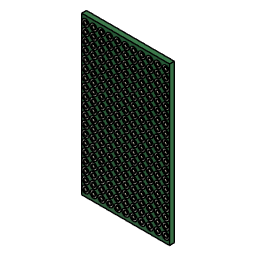
pcb_daughterboard (Autodesk Fusion 360 design; units mm, degrees)
Autodesk Fusion 360 part; units mm, degrees
(part 1 of 2)
sketch "PCB Daughterboard" plane through (0, 0, 0) normal (0, 1, 0) x (1, 0, 0)
  line L0 (0, 0) -> (38, 0)
  line L1 (38, 0) -> (38, -65)
  line L2 (38, -65) -> (0, -65)
  line L3 (0, -65) -> (0, 0)
  dimension "d3" = 38
  dimension "d4" = 65
  constraint horizontal L0
  constraint vertical L1
  constraint horizontal L2
  constraint vertical L3
  constraint coincident L0.start L3.end
  measures "d3" distance of L0.start L0.end
  measures "d4" distance of L0.end L1.end
extrude "Extrude1" add sketch "PCB Daughterboard" along normal blind 1.5 makes body 1
sketch "Holes" plane through (0, 0, 0) normal (0, -1, 0) x (1, 0, 0)
  line L0 (38, 65) -> (0, 65)
  line L1 (0, 65) -> (0, 0)
  line L2 (0, 0) -> (38, 0)
  line L3 (38, 0) -> (38, 65)
  circle A0 centre (1.22, 62.975) radius 0.6
  dimension "d5" = 1.2
  dimension "d12" = 1.22
  dimension "d13" = 2.025
  measures "d5" diameter of A0
  measures "d12" distance of L1 A0.centre
  measures "d13" distance of L0 A0.centre
extrude "Extrude2" cut sketch "Holes" against normal blind 1.5 contours A0 bodies 1
pattern_linear "R-Pattern1" count 19 spacing 2.5396 along (0, 0, -1) count 11 spacing 2.54 along (1, 0, 0) of "Extrude2"
sketch "Condutive Metal" plane through (0, 0, 0) normal (0, -1, 0) x (1, 0, 0)
  circle A0 centre (26.62, 17.262) radius 0.6
  circle A1 centre (26.62, 19.8016) radius 0.6
  circle A2 centre (26.62, 22.3412) radius 0.6
  circle A3 centre (26.62, 24.8808) radius 0.6
  circle A4 centre (26.62, 27.4204) radius 0.6
  circle A5 centre (26.62, 29.9601) radius 0.6
  circle A6 centre (26.62, 32.4997) radius 0.6
  circle A7 centre (26.62, 35.0393) radius 0.6
  circle A8 centre (26.62, 37.5789) radius 0.6
  circle A9 centre (26.62, 40.1185) radius 0.6
  circle A10 centre (26.62, 42.6581) radius 0.6
  circle A11 centre (26.62, 45.1977) radius 0.6
  circle A12 centre (26.62, 47.7373) radius 0.6
  circle A13 centre (26.62, 50.2769) radius 0.6
  circle A14 centre (26.62, 52.8166) radius 0.6
  circle A15 centre (26.62, 55.3562) radius 0.6
  circle A16 centre (26.62, 57.8958) radius 0.6
  circle A17 centre (26.62, 60.4354) radius 0.6
  circle A18 centre (26.62, 62.975) radius 0.6
  circle A19 centre (24.08, 17.262) radius 0.6
  circle A20 centre (24.08, 19.8016) radius 0.6
  circle A21 centre (24.08, 22.3412) radius 0.6
  circle A22 centre (24.08, 24.8808) radius 0.6
  circle A23 centre (24.08, 27.4204) radius 0.6
  circle A24 centre (24.08, 29.9601) radius 0.6
  circle A25 centre (24.08, 32.4997) radius 0.6
  circle A26 centre (24.08, 35.0393) radius 0.6
  circle A27 centre (24.08, 37.5789) radius 0.6
  circle A28 centre (24.08, 40.1185) radius 0.6
  circle A29 centre (24.08, 42.6581) radius 0.6
  circle A30 centre (24.08, 45.1977) radius 0.6
  circle A31 centre (24.08, 47.7373) radius 0.6
  circle A32 centre (24.08, 50.2769) radius 0.6
  circle A33 centre (24.08, 52.8166) radius 0.6
  circle A34 centre (24.08, 55.3562) radius 0.6
  circle A35 centre (24.08, 57.8958) radius 0.6
  circle A36 centre (24.08, 60.4354) radius 0.6
  circle A37 centre (24.08, 62.975) radius 0.6
  circle A38 centre (21.54, 17.262) radius 0.6
  circle A39 centre (21.54, 19.8016) radius 0.6
  circle A40 centre (21.54, 22.3412) radius 0.6
  circle A41 centre (21.54, 24.8808) radius 0.6
  circle A42 centre (21.54, 27.4204) radius 0.6
  circle A43 centre (21.54, 29.9601) radius 0.6
  circle A44 centre (21.54, 32.4997) radius 0.6
  circle A45 centre (21.54, 35.0393) radius 0.6
  circle A46 centre (21.54, 37.5789) radius 0.6
  circle A47 centre (21.54, 40.1185) radius 0.6
  circle A48 centre (21.54, 42.6581) radius 0.6
  circle A49 centre (21.54, 45.1977) radius 0.6
  circle A50 centre (21.54, 47.7373) radius 0.6
  circle A51 centre (21.54, 50.2769) radius 0.6
  circle A52 centre (21.54, 52.8166) radius 0.6
  circle A53 centre (21.54, 55.3562) radius 0.6
  circle A54 centre (21.54, 57.8958) radius 0.6
  circle A55 centre (21.54, 60.4354) radius 0.6
  circle A56 centre (21.54, 62.975) radius 0.6
  circle A57 centre (19, 17.262) radius 0.6
  circle A58 centre (19, 19.8016) radius 0.6
  circle A59 centre (19, 22.3412) radius 0.6
  circle A60 centre (19, 24.8808) radius 0.6
  circle A61 centre (19, 27.4204) radius 0.6
  circle A62 centre (19, 29.9601) radius 0.6
  circle A63 centre (19, 32.4997) radius 0.6
  circle A64 centre (19, 35.0393) radius 0.6
  circle A65 centre (19, 37.5789) radius 0.6
  circle A66 centre (19, 40.1185) radius 0.6
  circle A67 centre (19, 42.6581) radius 0.6
  circle A68 centre (19, 45.1977) radius 0.6
  circle A69 centre (19, 47.7373) radius 0.6
  circle A70 centre (19, 50.2769) radius 0.6
  circle A71 centre (19, 52.8166) radius 0.6
  circle A72 centre (19, 55.3562) radius 0.6
  circle A73 centre (19, 57.8958) radius 0.6
  circle A74 centre (19, 60.4354) radius 0.6
  circle A75 centre (19, 62.975) radius 0.6
  circle A76 centre (16.46, 17.262) radius 0.6
  circle A77 centre (16.46, 19.8016) radius 0.6
  circle A78 centre (16.46, 22.3412) radius 0.6
  circle A79 centre (16.46, 24.8808) radius 0.6
  circle A80 centre (16.46, 27.4204) radius 0.6
  circle A81 centre (16.46, 29.9601) radius 0.6
  circle A82 centre (16.46, 32.4997) radius 0.6
  circle A83 centre (16.46, 35.0393) radius 0.6
  circle A84 centre (16.46, 37.5789) radius 0.6
  circle A85 centre (16.46, 40.1185) radius 0.6
  circle A86 centre (16.46, 42.6581) radius 0.6
  circle A87 centre (16.46, 45.1977) radius 0.6
  circle A88 centre (16.46, 47.7373) radius 0.6
  circle A89 centre (16.46, 50.2769) radius 0.6
  circle A90 centre (16.46, 52.8166) radius 0.6
  circle A91 centre (16.46, 55.3562) radius 0.6
  circle A92 centre (16.46, 57.8958) radius 0.6
  circle A93 centre (16.46, 60.4354) radius 0.6
  circle A94 centre (16.46, 62.975) radius 0.6
  circle A95 centre (13.92, 17.262) radius 0.6
  circle A96 centre (13.92, 19.8016) radius 0.6
  circle A97 centre (13.92, 22.3412) radius 0.6
  circle A98 centre (13.92, 24.8808) radius 0.6
  circle A99 centre (13.92, 27.4204) radius 0.6
  circle A100 centre (13.92, 29.9601) radius 0.6
  circle A101 centre (13.92, 32.4997) radius 0.6
  circle A102 centre (13.92, 35.0393) radius 0.6
  circle A103 centre (13.92, 37.5789) radius 0.6
  circle A104 centre (13.92, 40.1185) radius 0.6
  circle A105 centre (13.92, 42.6581) radius 0.6
  circle A106 centre (13.92, 45.1977) radius 0.6
  circle A107 centre (13.92, 47.7373) radius 0.6
  circle A108 centre (13.92, 50.2769) radius 0.6
  circle A109 centre (13.92, 52.8166) radius 0.6
  circle A110 centre (13.92, 55.3562) radius 0.6
  circle A111 centre (13.92, 57.8958) radius 0.6
  circle A112 centre (13.92, 60.4354) radius 0.6
  circle A113 centre (13.92, 62.975) radius 0.6
  circle A114 centre (11.38, 17.262) radius 0.6
  circle A115 centre (11.38, 19.8016) radius 0.6
  circle A116 centre (11.38, 22.3412) radius 0.6
  circle A117 centre (11.38, 24.8808) radius 0.6
  circle A118 centre (11.38, 27.4204) radius 0.6
  circle A119 centre (11.38, 29.9601) radius 0.6
  circle A120 centre (11.38, 32.4997) radius 0.6
  circle A121 centre (11.38, 35.0393) radius 0.6
  circle A122 centre (11.38, 37.5789) radius 0.6
  circle A123 centre (11.38, 40.1185) radius 0.6
  circle A124 centre (11.38, 42.6581) radius 0.6
  circle A125 centre (11.38, 45.1977) radius 0.6
  circle A126 centre (11.38, 47.7373) radius 0.6
  circle A127 centre (11.38, 50.2769) radius 0.6
  circle A128 centre (11.38, 52.8166) radius 0.6
  circle A129 centre (11.38, 55.3562) radius 0.6
  circle A130 centre (11.38, 57.8958) radius 0.6
  circle A131 centre (11.38, 60.4354) radius 0.6
  circle A132 centre (11.38, 62.975) radius 0.6
  circle A133 centre (8.84, 17.262) radius 0.6
  circle A134 centre (8.84, 19.8016) radius 0.6
  circle A135 centre (8.84, 22.3412) radius 0.6
  circle A136 centre (8.84, 24.8808) radius 0.6
  circle A137 centre (8.84, 27.4204) radius 0.6
  circle A138 centre (8.84, 29.9601) radius 0.6
  circle A139 centre (8.84, 32.4997) radius 0.6
  circle A140 centre (8.84, 35.0393) radius 0.6
  circle A141 centre (8.84, 37.5789) radius 0.6
  circle A142 centre (8.84, 40.1185) radius 0.6
  circle A143 centre (8.84, 42.6581) radius 0.6
  circle A144 centre (8.84, 45.1977) radius 0.6
  circle A145 centre (8.84, 47.7373) radius 0.6
  circle A146 centre (8.84, 50.2769) radius 0.6
  circle A147 centre (8.84, 52.8166) radius 0.6
  circle A148 centre (8.84, 55.3562) radius 0.6
  circle A149 centre (8.84, 57.8958) radius 0.6
  circle A150 centre (8.84, 60.4354) radius 0.6
  circle A151 centre (8.84, 62.975) radius 0.6
  circle A152 centre (6.3, 17.262) radius 0.6
  circle A153 centre (6.3, 19.8016) radius 0.6
  circle A154 centre (6.3, 22.3412) radius 0.6
  circle A155 centre (6.3, 24.8808) radius 0.6
  circle A156 centre (6.3, 27.4204) radius 0.6
  circle A157 centre (6.3, 29.9601) radius 0.6
  circle A158 centre (6.3, 32.4997) radius 0.6
  circle A159 centre (6.3, 35.0393) radius 0.6
  circle A160 centre (6.3, 37.5789) radius 0.6
  circle A161 centre (6.3, 40.1185) radius 0.6
  circle A162 centre (6.3, 42.6581) radius 0.6
  circle A163 centre (6.3, 45.1977) radius 0.6
  circle A164 centre (6.3, 47.7373) radius 0.6
  circle A165 centre (6.3, 50.2769) radius 0.6
  circle A166 centre (6.3, 52.8166) radius 0.6
  circle A167 centre (6.3, 55.3562) radius 0.6
  circle A168 centre (6.3, 57.8958) radius 0.6
  circle A169 centre (6.3, 60.4354) radius 0.6
  circle A170 centre (6.3, 62.975) radius 0.6
  circle A171 centre (3.76, 17.262) radius 0.6
  circle A172 centre (3.76, 19.8016) radius 0.6
  circle A173 centre (3.76, 22.3412) radius 0.6
  circle A174 centre (3.76, 24.8808) radius 0.6
  circle A175 centre (3.76, 27.4204) radius 0.6
  circle A176 centre (3.76, 29.9601) radius 0.6
  circle A177 centre (3.76, 32.4997) radius 0.6
  circle A178 centre (3.76, 35.0393) radius 0.6
  circle A179 centre (3.76, 37.5789) radius 0.6
  circle A180 centre (3.76, 40.1185) radius 0.6
  circle A181 centre (3.76, 42.6581) radius 0.6
  circle A182 centre (3.76, 45.1977) radius 0.6
  circle A183 centre (3.76, 47.7373) radius 0.6
  circle A184 centre (3.76, 50.2769) radius 0.6
  circle A185 centre (3.76, 52.8166) radius 0.6
  circle A186 centre (3.76, 55.3562) radius 0.6
  circle A187 centre (3.76, 57.8958) radius 0.6
  circle A188 centre (3.76, 60.4354) radius 0.6
  circle A189 centre (3.76, 62.975) radius 0.6
  circle A190 centre (1.22, 17.262) radius 0.6
  circle A191 centre (1.22, 19.8016) radius 0.6
  circle A192 centre (1.22, 22.3412) radius 0.6
  circle A193 centre (1.22, 24.8808) radius 0.6
  circle A194 centre (1.22, 27.4204) radius 0.6
  circle A195 centre (1.22, 29.9601) radius 0.6
  circle A196 centre (1.22, 32.4997) radius 0.6
  circle A197 centre (1.22, 35.0393) radius 0.6
  circle A198 centre (1.22, 37.5789) radius 0.6
  circle A199 centre (1.22, 40.1185) radius 0.6
  circle A200 centre (1.22, 42.6581) radius 0.6
  circle A201 centre (1.22, 45.1977) radius 0.6
  circle A202 centre (1.22, 47.7373) radius 0.6
  circle A203 centre (1.22, 50.2769) radius 0.6
  circle A204 centre (1.22, 52.8166) radius 0.6
  circle A205 centre (1.22, 55.3562) radius 0.6
  circle A206 centre (1.22, 57.8958) radius 0.6
  circle A207 centre (1.22, 60.4354) radius 0.6
  circle A208 centre (1.22, 62.975) radius 0.6
  line L0 (38, 65) -> (0, 65)
  line L1 (0, 65) -> (0, 0)
  line L2 (0, 0) -> (38, 0)
  line L3 (38, 0) -> (38, 65)
  circle A209 centre (1.22, 62.975) radius 0.6
  circle A210 centre (1.22, 62.975) radius 1.1
  circle A211 centre (1.22, 62.975) radius 0.5
  dimension "d30" = 1.2
  dimension "d32" = 0.5
  dimension "d47" = 0.1
  constraint concentric A209 A210
  constraint concentric A209 A211
  measures "d30" diameter of A209
  measures "d32" distance of A209 A210
  measures "d47" distance of A209 A211
extrude "Extrude7" add sketch "Condutive Metal" against normal blind 1.5 separate body contours A208 A209 makes body 2
extrude "Extrude5" add sketch "Condutive Metal" along normal blind 0.01 separate body contours A208 A209 | A210 makes body 3
extrude "Extrude8" add sketch "Condutive Metal" against normal blind 0.01 from surface at -1.5 separate body contours A208 A209 | A210 makes body 4
pattern_linear "R-Pattern3" count 11 spacing 2.54 along (1, 0, 0) count 19 spacing 2.5396 along (0, 0, -1) of bodies 3 2 4 makes body 5 at (3.4863, 1, 63.5089) makes body 6 at (6.5468, 1, 62.4281) makes body 7 at (9.0868, 1, 63.5219) makes body 8 at (11.6268, 1, 63.5219) makes body 9 at (14.1668, 1, 63.5219) makes body 10 at (16.7068, 1, 63.5219) makes body 11 at (19.2468, 1, 63.5219) makes body 12 at (21.7868, 1, 63.5219) makes body 13 at (24.3268, 1, 63.5219) makes body 14 at (26.8668, 1, 63.5219) makes body 15 at (4.654, 0, 62.8955) makes body 16 at (7.194, 0, 62.8955) makes body 17 at (9.7359, 0, 62.9204) makes body 18 at (12.2759, 0, 62.9204) makes body 19 at (14.8159, 0, 62.9204) makes body 20 at (17.354, 0, 62.8955) makes body 21 at (19.894, 0, 62.8955) makes body 22 at (22.434, 0, 62.8955) makes body 23 at (24.974, 0, 62.8955) makes body 24 at (27.514, 0, 62.8955) makes body 25 at (4.654, 1.5, 62.8955) makes body 26 at (7.194, 1.5, 62.8955) makes body 27 at (9.7359, 1.5, 62.9204) makes body 28 at (12.2759, 1.5, 62.9204) makes body 29 at (14.8159, 1.5, 62.9204) makes body 30 at (17.354, 1.5, 62.8955) makes body 31 at (19.894, 1.5, 62.8955) makes body 32 at (22.434, 1.5, 62.8955) makes body 33 at (24.974, 1.5, 62.8955) makes body 34 at (27.514, 1.5, 62.8955) makes body 35 at (1.4668, 1, 60.9823) makes body 36 at (3.4863, 1, 60.9693) makes body 37 at (6.5468, 1, 59.8885) makes body 38 at (9.0868, 1, 60.9823) makes body 39 at (11.6268, 1, 60.9823) makes body 40 at (14.1668, 1, 60.9823) makes body 41 at (16.7068, 1, 60.9823) makes body 42 at (19.2468, 1, 60.9823) makes body 43 at (21.7868, 1, 60.9823) makes body 44 at (24.3268, 1, 60.9823) makes body 45 at (26.8668, 1, 60.9823) makes body 46 at (1.4668, 1, 58.4427) makes body 47 at (3.4863, 1, 58.4297) makes body 48 at (6.5468, 1, 57.3489) makes body 49 at (9.0868, 1, 58.4427) makes body 50 at (11.6268, 1, 58.4427) makes body 51 at (14.1668, 1, 58.4427) makes body 52 at (16.7068, 1, 58.4427) makes body 53 at (19.2468, 1, 58.4427) makes body 54 at (21.7868, 1, 58.4427) makes body 55 at (24.3268, 1, 58.4427) makes body 56 at (26.8668, 1, 58.4427) makes body 57 at (1.4668, 1, 55.9031) makes body 58 at (3.4863, 1, 55.8901) makes body 59 at (6.5468, 1, 54.8093) makes body 60 at (9.0868, 1, 55.9031) makes body 61 at (11.6268, 1, 55.9031) makes body 62 at (14.1668, 1, 55.9031) makes body 63 at (16.7068, 1, 55.9031) makes body 64 at (19.2468, 1, 55.9031) makes body 65 at (21.7868, 1, 55.9031) makes body 66 at (24.3268, 1, 55.9031) makes body 67 at (26.8668, 1, 55.9031) makes body 68 at (1.4668, 1, 53.3635) makes body 69 at (3.4863, 1, 53.3505) makes body 70 at (6.5468, 1, 52.2697) makes body 71 at (9.0868, 1, 53.3635) makes body 72 at (11.6268, 1, 53.3635) makes body 73 at (14.1668, 1, 53.3635) makes body 74 at (16.7068, 1, 53.3635) makes body 75 at (19.2468, 1, 53.3635) makes body 76 at (21.7868, 1, 53.3635) makes body 77 at (24.3268, 1, 53.3635) makes body 78 at (26.8668, 1, 53.3635) makes body 79 at (1.4668, 1, 50.8238) makes body 80 at (3.4863, 1, 50.8109) makes body 81 at (6.5468, 1, 49.73) makes body 82 at (9.0868, 1, 50.8238) makes body 83 at (11.6268, 1, 50.8238) makes body 84 at (14.1668, 1, 50.8238) makes body 85 at (16.7068, 1, 50.8238) makes body 86 at (19.2468, 1, 50.8238) makes body 87 at (21.7868, 1, 50.8238) makes body 88 at (24.3268, 1, 50.8238) makes body 89 at (26.8668, 1, 50.8238) makes body 90 at (1.4668, 1, 48.2842) makes body 91 at (3.4863, 1, 48.2713) makes body 92 at (6.5468, 1, 47.1904) makes body 93 at (9.0868, 1, 48.2842) makes body 94 at (11.6268, 1, 48.2842) makes body 95 at (14.1668, 1, 48.2842) makes body 96 at (16.7068, 1, 48.2842) makes body 97 at (19.2468, 1, 48.2842) makes body 98 at (21.7868, 1, 48.2842) makes body 99 at (24.3268, 1, 48.2842) makes body 100 at (26.8668, 1, 48.2842) makes body 101 at (1.4668, 1, 45.7446) makes body 102 at (3.4863, 1, 45.7316) makes body 103 at (6.5468, 1, 44.6508) makes body 104 at (9.0868, 1, 45.7446) makes body 105 at (11.6268, 1, 45.7446) makes body 106 at (14.1668, 1, 45.7446) makes body 107 at (16.7068, 1, 45.7446) makes body 108 at (19.2468, 1, 45.7446) makes body 109 at (21.7868, 1, 45.7446) makes body 110 at (24.3268, 1, 45.7446) makes body 111 at (26.8668, 1, 45.7446) makes body 112 at (1.4668, 1, 43.205) makes body 113 at (3.4863, 1, 43.192) makes body 114 at (6.5468, 1, 42.1112) makes body 115 at (9.0868, 1, 43.205) makes body 116 at (11.6268, 1, 43.205) makes body 117 at (14.1668, 1, 43.205) makes body 118 at (16.7068, 1, 43.205) makes body 119 at (19.2468, 1, 43.205) makes body 120 at (21.7868, 1, 43.205) makes body 121 at (24.3268, 1, 43.205) makes body 122 at (26.8668, 1, 43.205) makes body 123 at (1.4668, 1, 40.6654) makes body 124 at (3.4863, 1, 40.6524) makes body 125 at (6.5468, 1, 39.5716) makes body 126 at (9.0868, 1, 40.6654) makes body 127 at (11.6268, 1, 40.6654) makes body 128 at (14.1668, 1, 40.6654) makes body 129 at (16.7068, 1, 40.6654) makes body 130 at (19.2468, 1, 40.6654) makes body 131 at (21.7868, 1, 40.6654) makes body 132 at (24.3268, 1, 40.6654) makes body 133 at (26.8668, 1, 40.6654) makes body 134 at (1.4668, 1, 38.1258) makes body 135 at (3.4863, 1, 38.1128) makes body 136 at (6.5468, 1, 37.032) makes body 137 at (9.0868, 1, 38.1258) makes body 138 at (11.6268, 1, 38.1258) makes body 139 at (14.1668, 1, 38.1258) makes body 140 at (16.7068, 1, 38.1258) makes body 141 at (19.2468, 1, 38.1258) makes body 142 at (21.7868, 1, 38.1258) makes body 143 at (24.3268, 1, 38.1258) makes body 144 at (26.8668, 1, 38.1258) makes body 145 at (1.4668, 1, 35.5862) makes body 146 at (3.4863, 1, 35.5732) makes body 147 at (6.5468, 1, 34.4924) makes body 148 at (9.0868, 1, 35.5862) makes body 149 at (11.6268, 1, 35.5862) makes body 150 at (14.1668, 1, 35.5862) makes body 151 at (16.7068, 1, 35.5862) makes body 152 at (19.2468, 1, 35.5862) makes body 153 at (21.7868, 1, 35.5862) makes body 154 at (24.3268, 1, 35.5862) makes body 155 at (26.8668, 1, 35.5862) makes body 156 at (1.4668, 1, 33.0466) makes body 157 at (3.4863, 1, 33.0336) makes body 158 at (6.8993, 0.5, 32.5296) makes body 159 at (9.0868, 1, 33.0466) makes body 160 at (11.6268, 1, 33.0466) makes body 161 at (14.1668, 1, 33.0466) makes body 162 at (16.7068, 1, 33.0466) makes body 163 at (19.2468, 1, 33.0466) makes body 164 at (21.7868, 1, 33.0466) makes body 165 at (24.3268, 1, 33.0466) makes body 166 at (26.8668, 1, 33.0466) makes body 167 at (1.8193, 1, 29.9301) makes body 168 at (4.3593, 1, 29.9301) makes body 169 at (6.8993, 1, 29.9301) makes body 170 at (9.4393, 1, 29.9301) makes body 171 at (11.9793, 1, 29.9301) makes body 172 at (14.5193, 1, 29.9301) makes body 173 at (17.0593, 1, 29.9301) makes body 174 at (19.5993, 1, 29.9301) makes body 175 at (22.1393, 1, 29.9301) makes body 176 at (24.6793, 1, 29.9301) makes body 177 at (27.2193, 1, 29.9301) makes body 178 at (1.8193, 1, 27.3905) makes body 179 at (4.3593, 1, 27.3905) makes body 180 at (6.8993, 1, 27.3905) makes body 181 at (9.4393, 1, 27.3905) makes body 182 at (11.9793, 1, 27.3905) makes body 183 at (14.5193, 1, 27.3905) makes body 184 at (17.0593, 1, 27.3905) makes body 185 at (19.5993, 1, 27.3905) makes body 186 at (22.1393, 1, 27.3905) makes body 187 at (24.6793, 1, 27.3905) makes body 188 at (27.2193, 1, 27.3905) makes body 189 at (1.8193, 1, 24.8509) makes body 190 at (4.3593, 1, 24.8509) makes body 191 at (6.8993, 1, 24.8509) makes body 192 at (9.4393, 1, 24.8509) makes body 193 at (11.9793, 1, 24.8509) makes body 194 at (14.5193, 1, 24.8509) makes body 195 at (17.0593, 1, 24.8509) makes body 196 at (19.5993, 1, 24.8509) makes body 197 at (22.1393, 1, 24.8509) makes body 198 at (24.6793, 1, 24.8509) makes body 199 at (27.2193, 1, 24.8509) makes body 200 at (1.8193, 1, 22.3113) makes body 201 at (4.3593, 1, 22.3113) makes body 202 at (6.8993, 1, 22.3113) makes body 203 at (9.4393, 1, 22.3113) makes body 204 at (11.9793, 1, 22.3113) makes body 205 at (14.5193, 1, 22.3113) makes body 206 at (17.0593, 1, 22.3113) makes body 207 at (19.5993, 1, 22.3113) makes body 208 at (22.1393, 1, 22.3113) makes body 209 at (24.6793, 1, 22.3113) makes body 210 at (27.2193, 1, 22.3113) makes body 211 at (1.8193, 1, 19.7717) makes body 212 at (4.3593, 1, 19.7717) makes body 213 at (6.8993, 1, 19.7717) makes body 214 at (9.4393, 1, 19.7717) makes body 215 at (11.9793, 1, 19.7717) makes body 216 at (14.5193, 1, 19.7717) makes body 217 at (17.0593, 1, 19.7717) makes body 218 at (19.5993, 1, 19.7717) makes body 219 at (22.1393, 1, 19.7717) makes body 220 at (24.6793, 1, 19.7717) makes body 221 at (27.2193, 1, 19.7717) makes body 222 at (1.8193, 1, 17.2321) makes body 223 at (4.3593, 1, 17.2321) makes body 224 at (6.8993, 1, 17.2321) makes body 225 at (9.4393, 1, 17.2321) makes body 226 at (11.9793, 1, 17.2321) makes body 227 at (14.5193, 1, 17.2321) makes body 228 at (17.0593, 1, 17.2321) makes body 229 at (19.5993, 1, 17.2321) makes body 230 at (22.1393, 1, 17.2321) makes body 231 at (24.6793, 1, 17.2321) makes body 232 at (27.2193, 1, 17.2321) makes body 233 at (2.114, 0, 60.3559) makes body 234 at (4.654, 0, 60.3559) makes body 235 at (7.194, 0, 60.3559) makes body 236 at (9.7359, 0, 60.3807) makes body 237 at (12.2759, 0, 60.3807) makes body 238 at (14.8159, 0, 60.3807) makes body 239 at (17.354, 0, 60.3559) makes body 240 at (19.894, 0, 60.3559) makes body 241 at (22.434, 0, 60.3559) makes body 242 at (24.974, 0, 60.3559) makes body 243 at (27.514, 0, 60.3559) makes body 244 at (2.114, 0, 57.8163) makes body 245 at (4.654, 0, 57.8163) makes body 246 at (7.194, 0, 57.8163) makes body 247 at (9.7359, 0, 57.8411) makes body 248 at (12.2759, 0, 57.8411) makes body 249 at (14.8159, 0, 57.8411) makes body 250 at (17.354, 0, 57.8163) makes body 251 at (19.894, 0, 57.8163) makes body 252 at (22.434, 0, 57.8163) makes body 253 at (24.974, 0, 57.8163) makes body 254 at (27.514, 0, 57.8163) makes body 255 at (2.114, 0, 55.2767) makes body 256 at (4.654, 0, 55.2767) makes body 257 at (7.194, 0, 55.2767) makes body 258 at (9.7359, 0, 55.3015) makes body 259 at (12.2759, 0, 55.3015) makes body 260 at (14.8159, 0, 55.3015) makes body 261 at (17.354, 0, 55.2767) makes body 262 at (19.894, 0, 55.2767) makes body 263 at (22.434, 0, 55.2767) makes body 264 at (24.974, 0, 55.2767) makes body 265 at (27.514, 0, 55.2767) makes body 266 at (2.114, 0, 52.7371) makes body 267 at (4.654, 0, 52.7371) makes body 268 at (7.194, 0, 52.7371) makes body 269 at (9.734, 0, 52.7371) makes body 270 at (12.274, 0, 52.7371) makes body 271 at (14.814, 0, 52.7371) makes body 272 at (17.354, 0, 52.7371) makes body 273 at (19.894, 0, 52.7371) makes body 274 at (22.434, 0, 52.7371) makes body 275 at (24.974, 0, 52.7371) makes body 276 at (27.514, 0, 52.7371) makes body 277 at (2.114, 0, 50.1975) makes body 278 at (4.654, 0, 50.1975) makes body 279 at (7.194, 0, 50.1975) makes body 280 at (9.7359, 0, 50.2223) makes body 281 at (12.2759, 0, 50.2223) makes body 282 at (14.8159, 0, 50.2223) makes body 283 at (17.354, 0, 50.1975) makes body 284 at (19.894, 0, 50.1975) makes body 285 at (22.434, 0, 50.1975) makes body 286 at (24.974, 0, 50.1975) makes body 287 at (27.514, 0, 50.1975) makes body 288 at (2.114, 0, 47.6578) makes body 289 at (4.654, 0, 47.6578) makes body 290 at (7.194, 0, 47.6578) makes body 291 at (9.7359, 0, 47.6827) makes body 292 at (12.2759, 0, 47.6827) makes body 293 at (14.8159, 0, 47.6827) makes body 294 at (17.354, 0, 47.6578) makes body 295 at (19.894, 0, 47.6578) makes body 296 at (22.434, 0, 47.6578) makes body 297 at (24.974, 0, 47.6578) makes body 298 at (27.514, 0, 47.6578) makes body 299 at (2.114, 0, 45.1182) makes body 300 at (4.654, 0, 45.1182) makes body 301 at (7.194, 0, 45.1182) makes body 302 at (9.7359, 0, 45.1431) makes body 303 at (12.274, 0, 45.1182) makes body 304 at (14.814, 0, 45.1182) makes body 305 at (17.3559, 0, 45.1431) makes body 306 at (19.8959, 0, 45.1431) makes body 307 at (22.4359, 0, 45.1431) makes body 308 at (24.9759, 0, 45.1431) makes body 309 at (27.5159, 0, 45.1431) makes body 310 at (2.114, 0, 42.5786) makes body 311 at (4.654, 0, 42.5786) makes body 312 at (7.194, 0, 42.5786) makes body 313 at (9.7359, 0, 42.6035) makes body 314 at (12.2759, 0, 42.6035) makes body 315 at (14.8159, 0, 42.6035) makes body 316 at (17.354, 0, 42.5786) makes body 317 at (19.894, 0, 42.5786) makes body 318 at (22.434, 0, 42.5786) makes body 319 at (24.974, 0, 42.5786) makes body 320 at (27.514, 0, 42.5786) makes body 321 at (2.114, 0, 40.039) makes body 322 at (4.654, 0, 40.039) makes body 323 at (7.194, 0, 40.039) makes body 324 at (9.734, 0, 40.039) makes body 325 at (12.274, 0, 40.039) makes body 326 at (14.814, 0, 40.039) makes body 327 at (17.354, 0, 40.039) makes body 328 at (19.894, 0, 40.039) makes body 329 at (22.434, 0, 40.039) makes body 330 at (24.974, 0, 40.039) makes body 331 at (27.514, 0, 40.039) makes body 332 at (2.114, 0, 37.4994) makes body 333 at (4.654, 0, 37.4994) makes body 334 at (7.194, 0, 37.4994) makes body 335 at (9.7359, 0, 37.5242) makes body 336 at (12.2759, 0, 37.5242) makes body 337 at (14.8159, 0, 37.5242) makes body 338 at (17.354, 0, 37.4994) makes body 339 at (19.894, 0, 37.4994) makes body 340 at (22.434, 0, 37.4994) makes body 341 at (24.974, 0, 37.4994) makes body 342 at (27.514, 0, 37.4994) makes body 343 at (2.114, 0, 34.9598) makes body 344 at (4.654, 0, 34.9598) makes body 345 at (7.194, 0, 34.9598) makes body 346 at (9.7359, 0, 34.9846) makes body 347 at (12.2759, 0, 34.9846) makes body 348 at (14.8159, 0, 34.9846) makes body 349 at (17.354, 0, 34.9598) makes body 350 at (19.894, 0, 34.9598) makes body 351 at (22.434, 0, 34.9598) makes body 352 at (24.974, 0, 34.9598) makes body 353 at (27.514, 0, 34.9598) makes body 354 at (2.114, 0, 32.4202) makes body 355 at (4.654, 0, 32.4202) makes body 356 at (7.194, 0, 32.4202) makes body 357 at (9.734, 0, 32.4202) makes body 358 at (12.274, 0, 32.4202) makes body 359 at (14.814, 0, 32.4202) makes body 360 at (17.3559, 0, 32.445) makes body 361 at (19.8959, 0, 32.445) makes body 362 at (22.4359, 0, 32.445) makes body 363 at (24.9759, 0, 32.445) makes body 364 at (27.5159, 0, 32.445) makes body 365 at (2.114, 0, 29.8806) makes body 366 at (4.654, 0, 29.8806) makes body 367 at (7.194, 0, 29.8806) makes body 368 at (9.7359, 0, 29.9054) makes body 369 at (10.4841, 0, 29.9054) makes body 370 at (13.0241, 0, 29.9054) makes body 371 at (17.354, 0, 29.8806) makes body 372 at (18.1041, 0, 29.9054) makes body 373 at (20.6441, 0, 29.9054) makes body 374 at (23.1841, 0, 29.9054) makes body 375 at (25.7241, 0, 29.9054) makes body 376 at (2.114, 0, 27.341) makes body 377 at (4.654, 0, 27.341) makes body 378 at (7.194, 0, 27.341) makes body 379 at (9.7359, 0, 27.3658) makes body 380 at (10.4841, 0, 27.3658) makes body 381 at (13.0241, 0, 27.3658) makes body 382 at (17.354, 0, 27.341) makes body 383 at (18.1041, 0, 27.3658) makes body 384 at (20.6441, 0, 27.3658) makes body 385 at (23.1841, 0, 27.3658) makes body 386 at (25.7241, 0, 27.3658) makes body 387 at (2.114, 0, 24.8013) makes body 388 at (4.654, 0, 24.8013) makes body 389 at (7.194, 0, 24.8013) makes body 390 at (9.7359, 0, 24.8262) makes body 391 at (10.4841, 0, 24.8262) makes body 392 at (13.0241, 0, 24.8262) makes body 393 at (17.354, 0, 24.8013) makes body 394 at (18.1041, 0, 24.8262) makes body 395 at (20.6441, 0, 24.8262) makes body 396 at (23.1841, 0, 24.8262) makes body 397 at (25.7241, 0, 24.8262) makes body 398 at (2.114, 0, 22.2617) makes body 399 at (4.654, 0, 22.2617) makes body 400 at (7.194, 0, 22.2617) makes body 401 at (9.7359, 0, 22.2866) makes body 402 at (10.4841, 0, 22.2866) makes body 403 at (13.0241, 0, 22.2866) makes body 404 at (17.354, 0, 22.2617) makes body 405 at (18.1041, 0, 22.2866) makes body 406 at (20.6441, 0, 22.2866) makes body 407 at (23.1841, 0, 22.2866) makes body 408 at (25.7241, 0, 22.2866) makes body 409 at (2.114, 0, 19.7221) makes body 410 at (4.654, 0, 19.7221) makes body 411 at (7.194, 0, 19.7221) makes body 412 at (9.7359, 0, 19.747) makes body 413 at (10.4841, 0, 19.747) makes body 414 at (13.0241, 0, 19.747) makes body 415 at (17.354, 0, 19.7221) makes body 416 at (18.1041, 0, 19.747) makes body 417 at (20.6441, 0, 19.747) makes body 418 at (23.1841, 0, 19.747) makes body 419 at (25.7241, 0, 19.747) makes body 420 at (2.114, 0, 17.1825) makes body 421 at (4.654, 0, 17.1825) makes body 422 at (7.194, 0, 17.1825) makes body 423 at (9.7359, 0, 17.2074) makes body 424 at (10.4841, 0, 17.2074) makes body 425 at (13.0241, 0, 17.2074) makes body 426 at (17.354, 0, 17.1825) makes body 427 at (18.1041, 0, 17.2074) makes body 428 at (20.6441, 0, 17.2074) makes body 429 at (23.1841, 0, 17.2074) makes body 430 at (25.7241, 0, 17.2074) makes body 431 at (2.114, 1.5, 60.3559) makes body 432 at (4.654, 1.5, 60.3559) makes body 433 at (7.194, 1.5, 60.3559) makes body 434 at (9.7359, 1.5, 60.3807) makes body 435 at (12.2759, 1.5, 60.3807) makes body 436 at (14.8159, 1.5, 60.3807) makes body 437 at (17.354, 1.5, 60.3559) makes body 438 at (19.894, 1.5, 60.3559) makes body 439 at (22.434, 1.5, 60.3559) makes body 440 at (24.974, 1.5, 60.3559) makes body 441 at (27.514, 1.5, 60.3559) makes body 442 at (2.114, 1.5, 57.8163) makes body 443 at (4.654, 1.5, 57.8163) makes body 444 at (7.194, 1.5, 57.8163) makes body 445 at (9.7359, 1.5, 57.8411) makes body 446 at (12.2759, 1.5, 57.8411) makes body 447 at (14.8159, 1.5, 57.8411) makes body 448 at (17.354, 1.5, 57.8163) makes body 449 at (19.894, 1.5, 57.8163) makes body 450 at (22.434, 1.5, 57.8163) makes body 451 at (24.974, 1.5, 57.8163) makes body 452 at (27.514, 1.5, 57.8163) makes body 453 at (2.114, 1.5, 55.2767) makes body 454 at (4.654, 1.5, 55.2767) makes body 455 at (7.194, 1.5, 55.2767) makes body 456 at (9.7359, 1.5, 55.3015) makes body 457 at (12.2759, 1.5, 55.3015) makes body 458 at (14.8159, 1.5, 55.3015) makes body 459 at (17.354, 1.5, 55.2767) makes body 460 at (19.894, 1.5, 55.2767) makes body 461 at (22.434, 1.5, 55.2767) makes body 462 at (24.974, 1.5, 55.2767) makes body 463 at (27.514, 1.5, 55.2767) makes body 464 at (2.114, 1.5, 52.7371) makes body 465 at (4.654, 1.5, 52.7371) makes body 466 at (7.194, 1.5, 52.7371) makes body 467 at (9.734, 1.5, 52.7371) makes body 468 at (12.274, 1.5, 52.7371) makes body 469 at (14.814, 1.5, 52.7371) makes body 470 at (17.354, 1.5, 52.7371) makes body 471 at (19.894, 1.5, 52.7371) makes body 472 at (22.434, 1.5, 52.7371) makes body 473 at (24.974, 1.5, 52.7371) makes body 474 at (27.514, 1.5, 52.7371) makes body 475 at (2.114, 1.5, 50.1975) makes body 476 at (4.654, 1.5, 50.1975) makes body 477 at (7.194, 1.5, 50.1975) makes body 478 at (9.7359, 1.5, 50.2223) makes body 479 at (12.2759, 1.5, 50.2223) makes body 480 at (14.8159, 1.5, 50.2223) makes body 481 at (17.354, 1.5, 50.1975) makes body 482 at (19.894, 1.5, 50.1975) makes body 483 at (22.434, 1.5, 50.1975) makes body 484 at (24.974, 1.5, 50.1975) makes body 485 at (27.514, 1.5, 50.1975) makes body 486 at (2.114, 1.5, 47.6578) makes body 487 at (4.654, 1.5, 47.6578) makes body 488 at (7.194, 1.5, 47.6578) makes body 489 at (9.7359, 1.5, 47.6827) makes body 490 at (12.2759, 1.5, 47.6827) makes body 491 at (14.8159, 1.5, 47.6827) makes body 492 at (17.354, 1.5, 47.6578) makes body 493 at (19.894, 1.5, 47.6578) makes body 494 at (22.434, 1.5, 47.6578) makes body 495 at (24.974, 1.5, 47.6578) makes body 496 at (27.514, 1.5, 47.6578) makes body 497 at (2.114, 1.5, 45.1182) makes body 498 at (4.654, 1.5, 45.1182) makes body 499 at (7.194, 1.5, 45.1182) makes body 500 at (9.7359, 1.5, 45.1431) makes body 501 at (12.274, 1.5, 45.1182) makes body 502 at (14.814, 1.5, 45.1182) makes body 503 at (17.3559, 1.5, 45.1431) makes body 504 at (19.8959, 1.5, 45.1431) makes body 505 at (22.4359, 1.5, 45.1431) makes body 506 at (24.9759, 1.5, 45.1431) makes body 507 at (27.5159, 1.5, 45.1431) makes body 508 at (2.114, 1.5, 42.5786) makes body 509 at (4.654, 1.5, 42.5786) makes body 510 at (7.194, 1.5, 42.5786) makes body 511 at (9.7359, 1.5, 42.6035) makes body 512 at (12.2759, 1.5, 42.6035) makes body 513 at (14.8159, 1.5, 42.6035) makes body 514 at (17.354, 1.5, 42.5786) makes body 515 at (19.894, 1.5, 42.5786) makes body 516 at (22.434, 1.5, 42.5786) makes body 517 at (24.974, 1.5, 42.5786) makes body 518 at (27.514, 1.5, 42.5786) makes body 519 at (2.114, 1.5, 40.039) makes body 520 at (4.654, 1.5, 40.039) makes body 521 at (7.194, 1.5, 40.039) makes body 522 at (9.734, 1.5, 40.039) makes body 523 at (12.274, 1.5, 40.039) makes body 524 at (14.814, 1.5, 40.039) makes body 525 at (17.354, 1.5, 40.039) makes body 526 at (19.894, 1.5, 40.039) makes body 527 at (22.434, 1.5, 40.039) makes body 528 at (24.974, 1.5, 40.039) makes body 529 at (27.514, 1.5, 40.039) makes body 530 at (2.114, 1.5, 37.4994) makes body 531 at (4.654, 1.5, 37.4994) makes body 532 at (7.194, 1.5, 37.4994) makes body 533 at (9.7359, 1.5, 37.5242) makes body 534 at (12.2759, 1.5, 37.5242) makes body 535 at (14.8159, 1.5, 37.5242) makes body 536 at (17.354, 1.5, 37.4994) makes body 537 at (19.894, 1.5, 37.4994) makes body 538 at (22.434, 1.5, 37.4994) makes body 539 at (24.974, 1.5, 37.4994) makes body 540 at (27.514, 1.5, 37.4994) makes body 541 at (2.114, 1.5, 34.9598) makes body 542 at (4.654, 1.5, 34.9598) makes body 543 at (7.194, 1.5, 34.9598) makes body 544 at (9.7359, 1.5, 34.9846) makes body 545 at (12.2759, 1.5, 34.9846) makes body 546 at (14.8159, 1.5, 34.9846) makes body 547 at (17.354, 1.5, 34.9598) makes body 548 at (19.894, 1.5, 34.9598) makes body 549 at (22.434, 1.5, 34.9598) makes body 550 at (24.974, 1.5, 34.9598) makes body 551 at (27.514, 1.5, 34.9598) makes body 552 at (2.114, 1.5, 32.4202) makes body 553 at (4.654, 1.5, 32.4202) makes body 554 at (7.194, 1.5, 32.4202) makes body 555 at (9.734, 1.5, 32.4202) makes body 556 at (12.274, 1.5, 32.4202) makes body 557 at (14.814, 1.5, 32.4202) makes body 558 at (17.3559, 1.5, 32.445) makes body 559 at (19.8959, 1.5, 32.445) makes body 560 at (22.4359, 1.5, 32.445) makes body 561 at (24.9759, 1.5, 32.445) makes body 562 at (27.5159, 1.5, 32.445) makes body 563 at (2.114, 1.5, 29.8806) makes body 564 at (4.654, 1.5, 29.8806) makes body 565 at (7.194, 1.5, 29.8806) makes body 566 at (9.7359, 1.5, 29.9054) makes body 567 at (10.4841, 1.5, 29.9054) makes body 568 at (13.0241, 1.5, 29.9054) makes body 569 at (17.354, 1.5, 29.8806) makes body 570 at (18.1041, 1.5, 29.9054) makes body 571 at (20.6441, 1.5, 29.9054) makes body 572 at (23.1841, 1.5, 29.9054) makes body 573 at (25.7241, 1.5, 29.9054) makes body 574 at (2.114, 1.5, 27.341) makes body 575 at (4.654, 1.5, 27.341) makes body 576 at (7.194, 1.5, 27.341) makes body 577 at (9.7359, 1.5, 27.3658) makes body 578 at (10.4841, 1.5, 27.3658) makes body 579 at (13.0241, 1.5, 27.3658) makes body 580 at (17.354, 1.5, 27.341) makes body 581 at (18.1041, 1.5, 27.3658) makes body 582 at (20.6441, 1.5, 27.3658) makes body 583 at (23.1841, 1.5, 27.3658) makes body 584 at (25.7241, 1.5, 27.3658) makes body 585 at (2.114, 1.5, 24.8013) makes body 586 at (4.654, 1.5, 24.8013) makes body 587 at (7.194, 1.5, 24.8013) makes body 588 at (9.7359, 1.5, 24.8262) makes body 589 at (10.4841, 1.5, 24.8262) makes body 590 at (13.0241, 1.5, 24.8262) makes body 591 at (17.354, 1.5, 24.8013) makes body 592 at (18.1041, 1.5, 24.8262) makes body 593 at (20.6441, 1.5, 24.8262) makes body 594 at (23.1841, 1.5, 24.8262) makes body 595 at (25.7241, 1.5, 24.8262) makes body 596 at (2.114, 1.5, 22.2617) makes body 597 at (4.654, 1.5, 22.2617) makes body 598 at (7.194, 1.5, 22.2617) makes body 599 at (9.7359, 1.5, 22.2866) makes body 600 at (10.4841, 1.5, 22.2866) makes body 601 at (13.0241, 1.5, 22.2866) makes body 602 at (17.354, 1.5, 22.2617) makes body 603 at (18.1041, 1.5, 22.2866) makes body 604 at (20.6441, 1.5, 22.2866) makes body 605 at (23.1841, 1.5, 22.2866) makes body 606 at (25.7241, 1.5, 22.2866) makes body 607 at (2.114, 1.5, 19.7221) makes body 608 at (4.654, 1.5, 19.7221) makes body 609 at (7.194, 1.5, 19.7221) makes body 610 at (9.7359, 1.5, 19.747) makes body 611 at (10.4841, 1.5, 19.747) makes body 612 at (13.0241, 1.5, 19.747) makes body 613 at (17.354, 1.5, 19.7221) makes body 614 at (18.1041, 1.5, 19.747) makes body 615 at (20.6441, 1.5, 19.747) makes body 616 at (23.1841, 1.5, 19.747) makes body 617 at (25.7241, 1.5, 19.747) makes body 618 at (2.114, 1.5, 17.1825) makes body 619 at (4.654, 1.5, 17.1825) makes body 620 at (7.194, 1.5, 17.1825) makes body 621 at (9.7359, 1.5, 17.2074) makes body 622 at (10.4841, 1.5, 17.2074) makes body 623 at (13.0241, 1.5, 17.2074) makes body 624 at (17.354, 1.5, 17.1825) makes body 625 at (18.1041, 1.5, 17.2074) makes body 626 at (20.6441, 1.5, 17.2074) makes body 627 at (23.1841, 1.5, 17.2074) makes body 628 at (25.7241, 1.5, 17.2074)
sketch "Sketch6" plane through (0, 0, 0) normal (0, -1, 0) x (1, 0, 0)
  circle A0 centre (26.62, 17.262) radius 0.6
  circle A1 centre (26.62, 19.8016) radius 0.6
  circle A2 centre (26.62, 22.3412) radius 0.6
  circle A3 centre (26.62, 24.8808) radius 0.6
  circle A4 centre (26.62, 27.4204) radius 0.6
  circle A5 centre (26.62, 29.9601) radius 0.6
  circle A6 centre (26.62, 32.4997) radius 0.6
  circle A7 centre (26.62, 35.0393) radius 0.6
  circle A8 centre (26.62, 37.5789) radius 0.6
  circle A9 centre (26.62, 40.1185) radius 0.6
  circle A10 centre (26.62, 42.6581) radius 0.6
  circle A11 centre (26.62, 45.1977) radius 0.6
  circle A12 centre (26.62, 47.7373) radius 0.6
  circle A13 centre (26.62, 50.2769) radius 0.6
  circle A14 centre (26.62, 52.8166) radius 0.6
  circle A15 centre (26.62, 55.3562) radius 0.6
  circle A16 centre (26.62, 57.8958) radius 0.6
  circle A17 centre (26.62, 60.4354) radius 0.6
  circle A18 centre (26.62, 62.975) radius 0.6
  circle A19 centre (24.08, 17.262) radius 0.6
  circle A20 centre (24.08, 19.8016) radius 0.6
  circle A21 centre (24.08, 22.3412) radius 0.6
  circle A22 centre (24.08, 24.8808) radius 0.6
  circle A23 centre (24.08, 27.4204) radius 0.6
  circle A24 centre (24.08, 29.9601) radius 0.6
  circle A25 centre (24.08, 32.4997) radius 0.6
  circle A26 centre (24.08, 35.0393) radius 0.6
  circle A27 centre (24.08, 37.5789) radius 0.6
  circle A28 centre (24.08, 40.1185) radius 0.6
  circle A29 centre (24.08, 42.6581) radius 0.6
  circle A30 centre (24.08, 45.1977) radius 0.6
  circle A31 centre (24.08, 47.7373) radius 0.6
  circle A32 centre (24.08, 50.2769) radius 0.6
  circle A33 centre (24.08, 52.8166) radius 0.6
  circle A34 centre (24.08, 55.3562) radius 0.6
  circle A35 centre (24.08, 57.8958) radius 0.6
  circle A36 centre (24.08, 60.4354) radius 0.6
  circle A37 centre (24.08, 62.975) radius 0.6
  circle A38 centre (21.54, 17.262) radius 0.6
  circle A39 centre (21.54, 19.8016) radius 0.6
  circle A40 centre (21.54, 22.3412) radius 0.6
  circle A41 centre (21.54, 24.8808) radius 0.6
  circle A42 centre (21.54, 27.4204) radius 0.6
  circle A43 centre (21.54, 29.9601) radius 0.6
  circle A44 centre (21.54, 32.4997) radius 0.6
  circle A45 centre (21.54, 35.0393) radius 0.6
  circle A46 centre (21.54, 37.5789) radius 0.6
  circle A47 centre (21.54, 40.1185) radius 0.6
  circle A48 centre (21.54, 42.6581) radius 0.6
  circle A49 centre (21.54, 45.1977) radius 0.6
  circle A50 centre (21.54, 47.7373) radius 0.6
  circle A51 centre (21.54, 50.2769) radius 0.6
  circle A52 centre (21.54, 52.8166) radius 0.6
  circle A53 centre (21.54, 55.3562) radius 0.6
  circle A54 centre (21.54, 57.8958) radius 0.6
  circle A55 centre (21.54, 60.4354) radius 0.6
  circle A56 centre (21.54, 62.975) radius 0.6
  circle A57 centre (19, 17.262) radius 0.6
  circle A58 centre (19, 19.8016) radius 0.6
  circle A59 centre (19, 22.3412) radius 0.6
  circle A60 centre (19, 24.8808) radius 0.6
  circle A61 centre (19, 27.4204) radius 0.6
  circle A62 centre (19, 29.9601) radius 0.6
  circle A63 centre (19, 32.4997) radius 0.6
  circle A64 centre (19, 35.0393) radius 0.6
  circle A65 centre (19, 37.5789) radius 0.6
  circle A66 centre (19, 40.1185) radius 0.6
  circle A67 centre (19, 42.6581) radius 0.6
  circle A68 centre (19, 45.1977) radius 0.6
  circle A69 centre (19, 47.7373) radius 0.6
  circle A70 centre (19, 50.2769) radius 0.6
  circle A71 centre (19, 52.8166) radius 0.6
  circle A72 centre (19, 55.3562) radius 0.6
  circle A73 centre (19, 57.8958) radius 0.6
  circle A74 centre (19, 60.4354) radius 0.6
  circle A75 centre (19, 62.975) radius 0.6
  circle A76 centre (16.46, 17.262) radius 0.6
  circle A77 centre (16.46, 19.8016) radius 0.6
  circle A78 centre (16.46, 22.3412) radius 0.6
  circle A79 centre (16.46, 24.8808) radius 0.6
  circle A80 centre (16.46, 27.4204) radius 0.6
  circle A81 centre (16.46, 29.9601) radius 0.6
  circle A82 centre (16.46, 32.4997) radius 0.6
  circle A83 centre (16.46, 35.0393) radius 0.6
  circle A84 centre (16.46, 37.5789) radius 0.6
  circle A85 centre (16.46, 40.1185) radius 0.6
  circle A86 centre (16.46, 42.6581) radius 0.6
  circle A87 centre (16.46, 45.1977) radius 0.6
  circle A88 centre (16.46, 47.7373) radius 0.6
  circle A89 centre (16.46, 50.2769) radius 0.6
  circle A90 centre (16.46, 52.8166) radius 0.6
  circle A91 centre (16.46, 55.3562) radius 0.6
  circle A92 centre (16.46, 57.8958) radius 0.6
  circle A93 centre (16.46, 60.4354) radius 0.6
  circle A94 centre (16.46, 62.975) radius 0.6
  circle A95 centre (13.92, 17.262) radius 0.6
  circle A96 centre (13.92, 19.8016) radius 0.6
  circle A97 centre (13.92, 22.3412) radius 0.6
  circle A98 centre (13.92, 24.8808) radius 0.6
  circle A99 centre (13.92, 27.4204) radius 0.6
  circle A100 centre (13.92, 29.9601) radius 0.6
  circle A101 centre (13.92, 32.4997) radius 0.6
  circle A102 centre (13.92, 35.0393) radius 0.6
  circle A103 centre (13.92, 37.5789) radius 0.6
  circle A104 centre (13.92, 40.1185) radius 0.6
  circle A105 centre (13.92, 42.6581) radius 0.6
  circle A106 centre (13.92, 45.1977) radius 0.6
  circle A107 centre (13.92, 47.7373) radius 0.6
  circle A108 centre (13.92, 50.2769) radius 0.6
  circle A109 centre (13.92, 52.8166) radius 0.6
  circle A110 centre (13.92, 55.3562) radius 0.6
  circle A111 centre (13.92, 57.8958) radius 0.6
  circle A112 centre (13.92, 60.4354) radius 0.6
  circle A113 centre (13.92, 62.975) radius 0.6
  circle A114 centre (11.38, 17.262) radius 0.6
  circle A115 centre (11.38, 19.8016) radius 0.6
  circle A116 centre (11.38, 22.3412) radius 0.6
  circle A117 centre (11.38, 24.8808) radius 0.6
  circle A118 centre (11.38, 27.4204) radius 0.6
  circle A119 centre (11.38, 29.9601) radius 0.6
  circle A120 centre (11.38, 32.4997) radius 0.6
  circle A121 centre (11.38, 35.0393) radius 0.6
  circle A122 centre (11.38, 37.5789) radius 0.6
  circle A123 centre (11.38, 40.1185) radius 0.6
  circle A124 centre (11.38, 42.6581) radius 0.6
  circle A125 centre (11.38, 45.1977) radius 0.6
  circle A126 centre (11.38, 47.7373) radius 0.6
  circle A127 centre (11.38, 50.2769) radius 0.6
  circle A128 centre (11.38, 52.8166) radius 0.6
  circle A129 centre (11.38, 55.3562) radius 0.6
  circle A130 centre (11.38, 57.8958) radius 0.6
  circle A131 centre (11.38, 60.4354) radius 0.6
  circle A132 centre (11.38, 62.975) radius 0.6
  circle A133 centre (8.84, 17.262) radius 0.6
  circle A134 centre (8.84, 19.8016) radius 0.6
  circle A135 centre (8.84, 22.3412) radius 0.6
  circle A136 centre (8.84, 24.8808) radius 0.6
  circle A137 centre (8.84, 27.4204) radius 0.6
  circle A138 centre (8.84, 29.9601) radius 0.6
  circle A139 centre (8.84, 32.4997) radius 0.6
  circle A140 centre (8.84, 35.0393) radius 0.6
  circle A141 centre (8.84, 37.5789) radius 0.6
  circle A142 centre (8.84, 40.1185) radius 0.6
  circle A143 centre (8.84, 42.6581) radius 0.6
  circle A144 centre (8.84, 45.1977) radius 0.6
  circle A145 centre (8.84, 47.7373) radius 0.6
  circle A146 centre (8.84, 50.2769) radius 0.6
  circle A147 centre (8.84, 52.8166) radius 0.6
  circle A148 centre (8.84, 55.3562) radius 0.6
  circle A149 centre (8.84, 57.8958) radius 0.6
  circle A150 centre (8.84, 60.4354) radius 0.6
  circle A151 centre (8.84, 62.975) radius 0.6
  circle A152 centre (6.3, 17.262) radius 0.6
  circle A153 centre (6.3, 19.8016) radius 0.6
  circle A154 centre (6.3, 22.3412) radius 0.6
  circle A155 centre (6.3, 24.8808) radius 0.6
  circle A156 centre (6.3, 27.4204) radius 0.6
  circle A157 centre (6.3, 29.9601) radius 0.6
  circle A158 centre (6.3, 32.4997) radius 0.6
  circle A159 centre (6.3, 35.0393) radius 0.6
  circle A160 centre (6.3, 37.5789) radius 0.6
  circle A161 centre (6.3, 40.1185) radius 0.6
  circle A162 centre (6.3, 42.6581) radius 0.6
  circle A163 centre (6.3, 45.1977) radius 0.6
  circle A164 centre (6.3, 47.7373) radius 0.6
  circle A165 centre (6.3, 50.2769) radius 0.6
  circle A166 centre (6.3, 52.8166) radius 0.6
  circle A167 centre (6.3, 55.3562) radius 0.6
  circle A168 centre (6.3, 57.8958) radius 0.6
  circle A169 centre (6.3, 60.4354) radius 0.6
  circle A170 centre (6.3, 62.975) radius 0.6
  circle A171 centre (3.76, 17.262) radius 0.6
  circle A172 centre (3.76, 19.8016) radius 0.6
  circle A173 centre (3.76, 22.3412) radius 0.6
  circle A174 centre (3.76, 24.8808) radius 0.6
  circle A175 centre (3.76, 27.4204) radius 0.6
  circle A176 centre (3.76, 29.9601) radius 0.6
  circle A177 centre (3.76, 32.4997) radius 0.6
  circle A178 centre (3.76, 35.0393) radius 0.6
  circle A179 centre (3.76, 37.5789) radius 0.6
  circle A180 centre (3.76, 40.1185) radius 0.6
  circle A181 centre (3.76, 42.6581) radius 0.6
  circle A182 centre (3.76, 45.1977) radius 0.6
  circle A183 centre (3.76, 47.7373) radius 0.6
  circle A184 centre (3.76, 50.2769) radius 0.6
  circle A185 centre (3.76, 52.8166) radius 0.6
  circle A186 centre (3.76, 55.3562) radius 0.6
  circle A187 centre (3.76, 57.8958) radius 0.6
  circle A188 centre (3.76, 60.4354) radius 0.6
  circle A189 centre (3.76, 62.975) radius 0.6
  circle A190 centre (1.22, 17.262) radius 0.6
  circle A191 centre (1.22, 19.8016) radius 0.6
  circle A192 centre (1.22, 22.3412) radius 0.6
  circle A193 centre (1.22, 24.8808) radius 0.6
  circle A194 centre (1.22, 27.4204) radius 0.6
  circle A195 centre (1.22, 29.9601) radius 0.6
  circle A196 centre (1.22, 32.4997) radius 0.6
  circle A197 centre (1.22, 35.0393) radius 0.6
  circle A198 centre (1.22, 37.5789) radius 0.6
  circle A199 centre (1.22, 40.1185) radius 0.6
  circle A200 centre (1.22, 42.6581) radius 0.6
  circle A201 centre (1.22, 45.1977) radius 0.6
  circle A202 centre (1.22, 47.7373) radius 0.6
  circle A203 centre (1.22, 50.2769) radius 0.6
  circle A204 centre (1.22, 52.8166) radius 0.6
  circle A205 centre (1.22, 55.3562) radius 0.6
  circle A206 centre (1.22, 57.8958) radius 0.6
  circle A207 centre (1.22, 60.4354) radius 0.6
  circle A208 centre (1.22, 62.975) radius 0.6
  line L0 (38, 65) -> (0, 65)
  line L1 (0, 65) -> (0, 0)
  line L2 (0, 0) -> (38, 0)
  line L3 (38, 0) -> (38, 65)
  circle A209 centre (1.22, 62.975) radius 0.5
  circle A210 centre (1.22, 62.975) radius 1.1
  circle A211 centre (26.62, 62.975) radius 0.5
  circle A212 centre (26.62, 62.975) radius 1.1
  circle A213 centre (26.62, 17.262) radius 0.5
  circle A214 centre (26.62, 17.262) radius 1.1
  circle A215 centre (1.22, 17.262) radius 0.5
  circle A216 centre (1.22, 17.262) radius 1.1
  line L4 (38, 65) -> (27.84, 65)
  line L5 (27.84, 65) -> (27.84, 0)
  line L6 (27.84, 0) -> (38, 0)
  line L7 (38, 0) -> (38, 65)
  line L8 (0, 0) -> (27.84, 0)
  line L9 (27.84, 0) -> (27.84, 15.237)
  line L10 (27.84, 15.237) -> (0, 15.237)
  line L11 (0, 15.237) -> (0, 0)
  dimension "d48" = 2.025
  dimension "d49" = 1.22
  dimension "d50" = 1.22
  dimension "d51" = 2.025
  constraint horizontal L4
  constraint vertical L5
  constraint horizontal L6
  constraint vertical L7
  constraint coincident L2 L5.end
  constraint coincident L0.start L3.end
  constraint horizontal L8
  constraint vertical L9
  constraint horizontal L10
  constraint vertical L11
  constraint coincident L5 L9.end
  constraint coincident L1.end L2.start
  measures "d48" distance of A208.centre L0
  measures "d49" distance of A208.centre L1
  measures "d50" distance of A18.centre L5
  measures "d51" distance of A190.centre L10
extrude "Extrude9" cut sketch "Sketch6" against normal blind 1.5 contours L0 L2 L3 L4 L5 L6 L7 L9 | L1 L2 L5 L8 L9 L10 L11 bodies 1
equation "d12 = 0.72 mm + 0.5 mm"